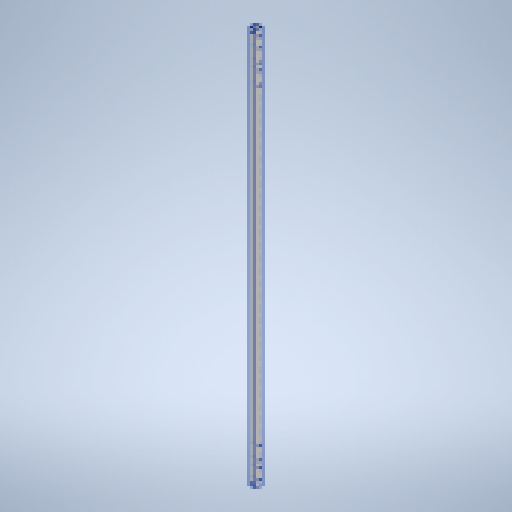
# Autodesk Inventor part: 10x10x600
Saved by Autodesk Inventor 2025 (Build 290162000, 162)
## iProperties
Created: 2025-02-24
Part Number: 10x10x600
Material: アルミニウム 6061
Document SubType Name: Modeling
Designer: Zhopa
Density: 2.7 g/cm^3
Appearance: アルミニウム - フラット
Mass: 57.8863 g
Surface Area: 431.613 cm^2
Volume: 21.4394 cm^3
Author: Zhopa
Autodesk Inventor part; units mm, degrees
ref_plane "YZ Plane" through (0, 0, 0) normal (1, 0, 0) x (0, 1, 0)
ref_plane "XZ Plane" through (0, 0, 0) normal (0, 1, 0) x (-1, 0, 0)
sketch "Sketch1" plane through (0, 0, 0) normal (0, 1, 0) x (-1, 0, 0)
  line L0 (-5, -5) -> (5, -5)
  line L1 (5, -5) -> (5, 5)
  line L2 (5, 5) -> (-5, 5)
  line L3 (-5, 5) -> (-5, -5)
  line L4 (-5, -5) -> (5, 5) construction
  line L5 (5, -5) -> (-5, 5) construction
  line L6 (-4, -4) -> (4, -4)
  line L7 (4, -4) -> (4, 4)
  line L8 (4, 4) -> (-4, 4)
  line L9 (-4, 4) -> (-4, -4)
  line L10 (-4, -4) -> (4, 4) construction
  line L11 (4, -4) -> (-4, 4) construction
  point P0 (0, 0)
  dimension "d0" = 10
  dimension "d1" = 10
  dimension "d2" = 8
  dimension "d3" = 8
  constraints: 24 end point, 4 midpoint, 4 parallel, 2 horizontal, 2 perpendicular
  measures "d0" distance of L2.end L1.end
  measures "d1" distance of L1.end L0.end
  measures "d2" distance of L8.end L7.end
  measures "d3" distance of L7.end L6.end
extrude "Extrusion1" add sketch "Sketch1" along normal blind 600
sketch "Sketch2" plane through (5, 0, -5) normal (1, 0, 0) x (0, 0, -1)
  line L0 (-10, 600) -> (0, 600) projected
  line L1 (-10, 0) -> (0, 0) projected
  point P0 (-5, 0)
  point P1 (-5, 545)
  point P2 (-5, 525)
  point P3 (-5, 590)
  point P4 (-5, 555)
  point P5 (-5, 575)
  point P6 (-5, 10)
  point P7 (-5, 25)
  point P8 (-5, 35)
  point P9 (-5, 55)
  point P10 (-5, 107.8006)
  dimension "d6" = 55
  dimension "d7" = 20
  dimension "d21" = 10
  dimension "d23" = 35
  dimension "d24" = 15
  dimension "d25" = 10
  dimension "d26" = 15
  dimension "d27" = 10
  dimension "d28" = 20
  measures "d6" distance from line of point (-5, 545) L0
  measures "d7" distance of point (-5, 525) point (-5, 545)
  measures "d21" distance from line of point (-5, 590) L0
  measures "d23" distance of point (-5, 555) point (-5, 590)
  measures "d24" distance of point (-5, 575) point (-5, 590)
  measures "d25" distance from line of L1 point (-5, 10)
  measures "d26" distance of point (-5, 10) point (-5, 25)
  measures "d27" distance of point (-5, 25) point (-5, 35)
  measures "d28" distance of point (-5, 35) point (-5, 55)
hole "Hole1" at (5, 545, 0) at (5, 525, 0) at (5, 590, 0) at (5, 555, 0) at (5, 575, 0) at (5, 10, 0) at (5, 25, 0) at (5, 35, 0) at (5, 55, 0) direction (-1, 0, 0) diameter 3 depth 80.45
sketch "Sketch3" plane through (-5, 0, -5) normal (0, 0, -1) x (-1, 0, 0)
  line L0 (-10, 600) -> (0, 600) projected
  circle A0 centre (-5, 595) radius 1.5
  line L1 (-10, 0) -> (0, 0) projected
  circle A1 centre (-5, 5) radius 1.75
  point P0 (-5, 0)
  dimension "d15" = 5
  dimension "d16" = 3
  dimension "d19" = 5
  dimension "d20" = 3.5
  constraints: 2 centre point, 2 coincident
  measures "d15" distance from line of point (-5, 595) L0
  measures "d16" diameter of A0
  measures "d19" distance from line of L1 point (-5, 5)
  measures "d20" diameter of A1
extrude "Extrusion2" cut sketch "Sketch3" against normal blind 600
ref_plane "Work Plane1" through (0, 300, 0) normal (0, 1, 0) x (1, 0, 0)
body "Solid1"
